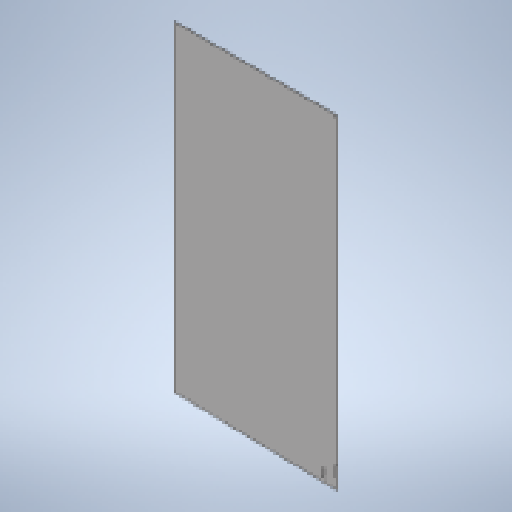
# Autodesk Inventor part: GBK 2211 shield 4
Saved by Autodesk Inventor 2026 (Build 300175000, 175)
## iProperties
Created: 2026-04-17
Part Number: GBK 2211 shield 4
Material: Steel
Document SubType Name: Sheet Metal
Designer: pokla
Stock Number: 2214
Mass: 138487 g
Surface Area: 88564.8 cm^2
Volume: 17641.6 cm^3
Density: 7.85 g/cm^3
Flat Pattern Width: 148 cm
Flat Pattern Length: 292 cm
Flat Pattern Area: 43216 cm^2
Sheet Metal Rule: По умолчанию_мм
Sheet Metal Width: 1480,000 мм
Sheet Metal Length: 2920,000 мм
Sheet Metal Area: 4321600,000 мм^2
Appearance: Default
Author: admin
Autodesk Inventor part; units mm, degrees
ref_plane "YZ Plane" through (0, 0, 0) normal (1, 0, 0) x (0, 1, 0)
ref_plane "XZ Plane" through (0, 0, 0) normal (0, 1, 0) x (-1, 0, 0)
ref_plane "XY Plane" through (0, 0, 0) normal (0, 0, 1) x (1, 0, 0)
sketch "Sketch1" plane through (0, 0, 0) normal (0, 0, 1) x (1, 0, 0)
  line L0 (740, -1490) -> (-740, -1490)
  line L1 (-740, -1490) -> (-740, 1490)
  line L2 (-740, 1490) -> (740, 1490)
  line L3 (740, 1490) -> (740, -1490)
  line L4 (740, -1490) -> (-740, 1490) construction
  line L5 (-740, -1490) -> (740, 1490) construction
  line L6 (740, -1430) -> (-740, -1396.4141)
  point P0 (0, 0)
  dimension "d0" = 1480
  dimension "d1" = 2980
  dimension "d3" = 1.3
  dimension "d4" = 60
  measures "d0" distance of L1.end L2.end
  measures "d1" distance of L0.end L1.end
  measures "d3" angle of L0 L6
  measures "d4" distance of L0.start L6.start
extrude "Plate1" add sketch "Sketch1" along normal blind 4 contours L6 L1 L2 L3
sketch "Sketch2" plane through (0, 0, 4) normal (0, 0, 1) x (1, 0, 0)
  line L0 (621.6658, -1316.5027) -> (621.6658, -1674.1932) construction
  line L1 (621.6658, -1674.1932) -> (530.4095, -1674.1932) construction
  line L2 (530.4095, -1674.1932) -> (530.4095, -1316.5027) construction
  line L3 (530.4095, -1316.5027) -> (621.6658, -1316.5027) construction
  line L4 (770, -1236) -> (710, -1236) projected
  line L5 (710, -1240) -> (710, -1236) projected
  line L6 (710.2537, -1243.5) -> (710.2537, -1340.5) projected
  line L7 (710.2537, -1340.5) -> (706.2547, -1340.5) projected
  ellipse E0 centre (710.2537, 1484.5) end of major axis (710.2537, 1514.5) minor radius 0.6803 (710.2537, 1454.5) -> (710.2537, 1514.5) ccw projected
  line L8 (710.2537, 1454.5) -> (706.2547, 1454.5) projected
  line L9 (770, 1247.3333) -> (710, 1247.3333) projected
  line L10 (710, 1243.3333) -> (710, 1247.3333) projected
  line L11 (770, 750.6667) -> (710, 750.6667) projected
  line L12 (710, 746.6667) -> (710, 750.6667) projected
  line L13 (770, 254) -> (710, 254) projected
  line L14 (710, 250) -> (710, 254) projected
  line L15 (770, -242.6667) -> (710, -242.6667) projected
  line L16 (710, -246.6667) -> (710, -242.6667) projected
  line L17 (770, -739.3333) -> (710, -739.3333) projected
  line L18 (710, -743.3333) -> (710, -739.3333) projected
  ellipse E1 centre (210.1251, 1484.5) end of major axis (210.1251, 1514.5) minor radius 0.6803 (210.1251, 1454.5) -> (210.1251, 1514.5) ccw projected
  line L19 (210.1251, 1454.5) -> (206.1261, 1454.5) projected
  ellipse E2 centre (-290.0035, 1484.5) end of major axis (-290.0035, 1514.5) minor radius 0.6803 (-290.0035, 1454.5) -> (-290.0035, 1514.5) ccw projected
  line L20 (-290.0035, 1454.5) -> (-294.0025, 1454.5) projected
  line L21 (-710, 1247.3333) -> (-739.3197, 1247.3333) projected
  line L22 (-710, 1243.3333) -> (-710, 1247.3333) projected
  line L23 (-710, 750.6667) -> (-739.3197, 750.6667) projected
  line L24 (-710, 746.6667) -> (-710, 750.6667) projected
  line L25 (-710, 254) -> (-739.3197, 254) projected
  line L26 (-710, 250) -> (-710, 254) projected
  line L27 (-710, -242.6667) -> (-739.3197, -242.6667) projected
  line L28 (-710, -246.6667) -> (-710, -242.6667) projected
  line L29 (-710, -739.3333) -> (-739.3197, -739.3333) projected
  line L30 (-710, -743.3333) -> (-710, -739.3333) projected
  line L31 (-710, -1236) -> (-739.3197, -1236) projected
  line L32 (-710, -1240) -> (-710, -1236) projected
  line L33 (-290.0035, -1243.5) -> (-290.0035, -1340.5) projected
  line L34 (-290.0035, -1340.5) -> (-294.0025, -1340.5) projected
  line L35 (210.1251, -1243.5) -> (210.1251, -1340.5) projected
  line L36 (210.1251, -1340.5) -> (206.1261, -1340.5) projected
  point P0 (0, 0)
  constraints: 5 other
mark "Mark1"
equation "\"d0\" = Лист_ширина"
equation "\"d2\" = Thickness"
equation "\"BendRadius\" = Thickness"
equation "\"BendReliefWidth\" = Thickness"
equation "\"BendReliefDepth\" = 0.5 * Thickness"
equation "\"CornerReliefSize\" = 4 * Thickness"
equation "\"MinimumRemnant\" = 2 * Thickness"
equation "\"TransitionRadius\" = BendRadius"
equation "\"JacobiRadiusSize\" = BendRadius"
equation "\"GapSize\" = Thickness"
equation "\"Лист_ширина\" = 1480"
equation "\"Thickness\" = 4"
body "Solid1"
